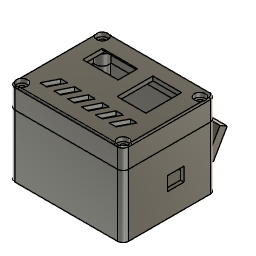
CaseCameraSlider (Autodesk Fusion 360 design; units mm, degrees)
Autodesk Fusion 360 part; units mm, degrees
note: some values were not read from the file. Set by a fixed rule: which face or edge a step refers to.
sketch "Schizzo3" plane through (0, 0, 0) normal (0, 0, 1) x (1, 0, 0)
  line L0 (0, 0) -> (80, 0)
  line L1 (80, 0) -> (80, -65)
  line L2 (80, -65) -> (0, -65)
  line L3 (0, -65) -> (0, 0)
  line L4 (81, -66) -> (-1, -66)
  line L5 (-1, -66) -> (-1, 1)
  line L6 (-1, 1) -> (81, 1)
  line L7 (81, 1) -> (81, -66)
  dimension "d8" = 80
  dimension "d9" = 65
  dimension "d10" = -1
  constraint horizontal L0
  constraint vertical L1
  constraint horizontal L2
  constraint vertical L3
  constraint coincident L0.start L3.end
  measures "d8" distance of L0.start L0.end
  measures "d9" distance of L0.start L2.end
extrude "Estrusione2" add sketch "Schizzo3" along normal blind 60 contours L0 L1 L2 L3 | L4 L5 L6 L7 makes body 1
sketch "Schizzo9" plane through (0, 0, 60) normal (0, 0, 1) x (-1, 0, 0)
  line L0 (-81, -1) -> (1, -1)
  line L1 (1, -1) -> (1, 66)
  line L2 (1, 66) -> (-81, 66)
  line L3 (-81, 66) -> (-81, -1)
  line L4 (1, -1) -> (-3.5, -1)
  line L5 (-3.5, -1) -> (-3.5, 3.5)
  line L6 (-3.5, 3.5) -> (1, 3.5)
  line L7 (1, 3.5) -> (1, -1)
  circle A0 centre (-3.5, 3.5) radius 4
  circle A1 centre (-3.5, 3.5) radius 2
  circle A2 centre (-76.5, 6.0015) radius 2
  circle A3 centre (-76.5, 6.0015) radius 4
  circle A4 centre (-3.5, 61.5) radius 2
  circle A5 centre (-3.5, 61.5) radius 4
  circle A6 centre (-76.5, 61.5) radius 2
  circle A7 centre (-76.5, 61.5) radius 4
  dimension "d70" = 4.5
  dimension "d71" = 4.5
  dimension "d72" = 8
  dimension "d73" = 4
  dimension "d81" = 8
  dimension "d82" = 4
  dimension "d86" = 8
  dimension "d87" = 4
  dimension "d88" = 8
  dimension "d89" = 4
  dimension "d90" = 4.5
  dimension "d91" = 4.5
  dimension "d92" = 4.5
  dimension "d93" = 4.5
  dimension "d94" = 4.5
  dimension "d95" = 4.5
  dimension "d96" = 4.5
  dimension "d97" = 4.5
  dimension "d98" = 4.5
  constraint horizontal L4
  constraint vertical L5
  constraint horizontal L6
  constraint vertical L7
  constraint coincident L0.end L1.start
  constraint coincident L5.end L6.start
  constraint concentric A0 A1
  constraint concentric A2 A3
  measures "d70" distance of L0.end L4.end
  measures "d71" distance of L0.end L6.end
  measures "d72" diameter of A0
  measures "d73" diameter of A1
  measures "d81" diameter of A3
  measures "d82" diameter of A2
  measures "d86" diameter of A5
  measures "d87" diameter of A4
  measures "d88" diameter of A7
  measures "d89" diameter of A6
  measures "d90" distance of L1 A4.centre
  measures "d91" distance of L1 A4.centre
  measures "d92" distance of L2 A4.centre
  measures "d93" distance of L2 A4.centre
  measures "d94" distance of L3 A2.centre
  measures "d95" distance of L3 A6.centre
  measures "d96" distance of L3 A6.centre
  measures "d97" distance of L2 A6.centre
  measures "d98" distance of L2 A6.centre
extrude "Estrusione9" cut sketch "Schizzo9" against normal blind 3 contours A3 bodies 1
extrude "Estrusione7" cut sketch "Schizzo9" against normal blind 3 contours L5 L6 A0 A1 | L5 L6 A0 A1 bodies 1
extrude "Estrusione8" cut 1 faces at (4.6392, -4.0006, 60) along direction (0, 0, -1) blind 20 on bodies 1 bodies 1
extrude "Estrusione10" cut sketch "Schizzo9" against normal blind 20 contours A2 bodies 1
extrude "Estrusione11" cut sketch "Schizzo9" against normal blind 3 contours A7 bodies 1
extrude "Estrusione12" cut sketch "Schizzo9" against normal blind 20 contours A6 bodies 1
extrude "Estrusione13" cut sketch "Schizzo9" against normal blind 3 contours A5 bodies 1
extrude "Estrusione14" cut sketch "Schizzo9" against normal blind 20 contours A4 bodies 1
fillet "Raccordo2" radius 4 4 edges at (-1, -66, 30) (81, -66, 30) (-1, 1, 30) (81, 1, 30) on bodies 1
ref_plane "Piano di lavoro2" through (40, -32.5, 45) normal (0, 0, 1) x (1, 0, 0)
split "Dividi2" by plane through (40, -32.5, 45) normal (0, 0, 1) bodies 1 makes body 2 at (28.6865, -24.4183, 60)
shell "Shell3" thickness 2.5 removed faces 1 at (28.2599, -24.0427, 45) on bodies 1
shell "Shell4" thickness 3 removed faces 1 at (28.2599, -24.0427, 45) on bodies 2
fillet "Raccordo3" radius 1 8 edges at (0.1716, -64.8284, 60) (-1, -32.5, 60) (0.1716, -0.1716, 60) (40, 1, 60) (79.8284, -0.1716, 60) (81, -32.5, 60) (79.8284, -64.8284, 60) (40, -66, 60) on bodies 2
sketch "Schizzo20" plane through (0, 1, 0) normal (0, 1, 0) x (-1, 0, 0)
  line L0 (-3, 45) -> (-77, 45)
  line L1 (-77, 45) -> (-77, 0)
  line L2 (-77, 0) -> (-3, 0)
  line L3 (-3, 0) -> (-3, 45)
  line L4 (-50, 22.0662) -> (-25, 22.0662)
  line L5 (-25, 22.0662) -> (-25, 12.0662)
  line L6 (-25, 12.0662) -> (-50, 12.0662)
  line L7 (-50, 12.0662) -> (-50, 22.0662)
  dimension "d178" = 10
  constraint horizontal L4
  constraint vertical L5
  constraint horizontal L6
  constraint vertical L7
  measures "d178" distance of L4.start L6.end
extrude "Estrusione28" add sketch "Schizzo20" along normal blind 15 contours L4 L5 L6 L7 bodies 1
sketch "Schizzo21" plane through (50, 0, 0) normal (1, 0, 0) x (0, 1, 0)
  line L0 (1, 22.0662) -> (1, 12.0662)
  line L1 (1, 12.0662) -> (16, 12.0662)
  line L2 (16, 12.0662) -> (16, 22.0662)
  line L3 (16, 22.0662) -> (1, 22.0662)
  line L4 (16, 22.0662) -> (10.2265, 12.0662)
  line L5 (16, 22.0662) -> (27.547, 22.0662) construction
  dimension "d325" = 120
  constraint horizontal L5
  constraint coincident L2.end L3.start
  constraint coincident L1 L4.end
  measures "d325" angle of L4 L5
extrude "Estrusione29" cut sketch "Schizzo21" against normal up to surface (25 mm away) contours L1 L2 L4 bodies 1
sketch "Schizzo28" plane through (0, 1, 0) normal (0, 1, 0) x (-1, 0, 0)
  line L0 (-70, 25) -> (-63, 25)
  line L1 (-63, 25) -> (-63, 15)
  line L2 (-63, 15) -> (-70, 15)
  line L3 (-70, 15) -> (-70, 25)
  dimension "d197" = 7
  dimension "d202" = 10
  constraint horizontal L0
  constraint vertical L1
  constraint horizontal L2
  constraint vertical L3
  measures "d197" distance of L0.start L0.end
  measures "d202" distance of L0.start L2.end
extrude "Estrusione35" cut sketch "Schizzo28" against normal up to surface (2.5 mm away) bodies 1
fillet "Raccordo11" radius 2 4 edges at (63, -0.25, 15) (70, -0.25, 15) (63, -0.25, 25) (70, -0.25, 25) on bodies 1
sketch "Schizzo34" plane through (0, 0, 2.5) normal (0, 0, 1) x (-1, 0, 0)
  arc A0 (-78.5, 3) -> (-77, 1.5) centre (-77, 3) ccw
  line L0 (-77, 1.5) -> (-3, 1.5)
  arc A1 (-3, 1.5) -> (-1.5, 3) centre (-3, 3) ccw
  line L1 (-1.5, 3) -> (-1.5, 62)
  arc A2 (-1.5, 62) -> (-3, 63.5) centre (-3, 62) ccw
  line L2 (-3, 63.5) -> (-77, 63.5)
  arc A3 (-77, 63.5) -> (-78.5, 62) centre (-77, 62) ccw
  line L3 (-78.5, 62) -> (-78.5, 3)
  line L4 (-75, 1.5) -> (-3, 1.5)
  line L5 (-76, 64) -> (-4, 64)
  circle A4 centre (-22.5, 6) radius 1.5
  circle A5 centre (-72, 6) radius 1.5
  circle A6 centre (-72, 58.5) radius 1.5
  circle A7 centre (-72, 36.5) radius 1.5
  circle A8 centre (-6, 58.5) radius 1.5
  circle A9 centre (-6, 58.5) radius 3
  circle A10 centre (-72, 58.5) radius 3
  circle A11 centre (-72, 36.5) radius 3
  circle A12 centre (-72, 6) radius 3
  circle A13 centre (-22.5, 6) radius 3
  point P0 (-40, 34.5)
  dimension "d274" = 72
  dimension "d279" = 3
  dimension "d280" = 3
  dimension "d281" = 3
  dimension "d282" = 3
  dimension "d283" = 3
  dimension "d294" = 6
  dimension "d295" = 6
  dimension "d296" = 6
  dimension "d297" = 6
  dimension "d298" = 6
  constraint horizontal L5
  constraint concentric A8 A9
  constraint concentric A6 A10
  constraint concentric A7 A11
  constraint concentric A5 A12
  constraint concentric A4 A13
  measures "d274" distance of L4.start L0.end
  measures "d279" diameter of A4
  measures "d280" diameter of A5
  measures "d281" diameter of A6
  measures "d282" diameter of A7
  measures "d283" diameter of A8
  measures "d294" diameter of A9
  measures "d295" diameter of A10
  measures "d296" diameter of A11
  measures "d297" diameter of A12
  measures "d298" diameter of A13
extrude "Estrusione48" add sketch "Schizzo34" along normal blind 4 contours A9 | A10 | A11 | A12 | A13 bodies 1
sketch "Schizzo35" plane through (1.5, 0, 0) normal (1, 0, 0) x (0, 1, 0)
  line L0 (-57.4689, 45) -> (-57.4689, 37.5)
  line L1 (-57.4689, 37.5) -> (-62, 37.5)
  line L2 (-62, 37.5) -> (-62, 2.5)
  line L3 (-62, 2.5) -> (-3, 2.5)
  line L4 (-3, 2.5) -> (-3, 37.5)
  line L5 (-3, 37.5) -> (-7.5311, 37.5)
  line L6 (-7.5311, 37.5) -> (-7.5311, 45)
  line L7 (-7.5311, 45) -> (-57.4689, 45)
sketch "Schizzo36" plane through (-1, 0, 0) normal (-1, 0, 0) x (0, -1, 0)
  line L0 (62, 45) -> (3, 45)
  line L1 (3, 45) -> (3, 0)
  line L2 (3, 0) -> (62, 0)
  line L3 (62, 0) -> (62, 45)
  line L4 (5, 16.5) -> (15, 16.5)
  line L5 (15, 16.5) -> (15, 6.5)
  line L6 (15, 6.5) -> (5, 6.5)
  line L7 (5, 6.5) -> (5, 16.5)
  point P0 (32.5, 23.8824)
  dimension "d305" = 10
  dimension "d306" = 10
  dimension "d324" = 2
  constraint horizontal L4
  constraint vertical L5
  constraint horizontal L6
  constraint vertical L7
  measures "d305" distance of L4.start L4.end
  measures "d306" distance of L4.start L6.end
  measures "d324" distance of L1 L7
extrude "Estrusione49" cut sketch "Schizzo36" against normal blind 2.5 contours L4 L5 L6 L7 bodies 1
sketch "Schizzo41" plane through (81, 0, 0) normal (1, 0, 0) x (0, 1, 0)
  line L0 (-3, 45) -> (-62, 45)
  line L1 (-62, 45) -> (-62, 0)
  line L2 (-62, 0) -> (-3, 0)
  line L3 (-3, 0) -> (-3, 45)
  line L4 (-22, 17) -> (-34, 17)
  line L5 (-34, 17) -> (-34, 27)
  line L6 (-34, 27) -> (-22, 27)
  line L7 (-22, 27) -> (-22, 17)
  point P0 (-28, 22)
  dimension "d312" = 12
  dimension "d313" = 10
  dimension "d315" = 18
  dimension "d316" = 25
  constraint horizontal L4
  constraint vertical L5
  constraint horizontal L6
  constraint vertical L7
  measures "d312" distance of L4.start L4.end
  measures "d313" distance of L4.start L6.end
  measures "d315" distance of L0 L6
  measures "d316" distance of L3 P0
extrude "Estrusione50" cut sketch "Schizzo41" against normal up to surface (2.5 mm away) contours L4 L5 L6 L7 bodies 1
sketch "Schizzo43" plane through (0, 2.445, -1.4116) normal (0, 0.866025, -0.5) x (-1, 0, 0)
  line L0 (-25, 15.5629) -> (-25, 27.1099)
  line L1 (-25, 27.1099) -> (-50, 27.1099)
  line L2 (-50, 27.1099) -> (-50, 15.5629)
  line L3 (-50, 15.5629) -> (-25, 15.5629)
  line L4 (-7, 11) -> (-67, 11)
  line L5 (-67, 11) -> (-67, 31)
  line L6 (-67, 31) -> (-7, 31)
  line L7 (-7, 31) -> (-7, 11)
  line L8 (-7, 11) -> (-67, 31) construction
  line L9 (-67, 11) -> (-7, 31) construction
  point P0 (-37, 21)
  dimension "d326" = 60
  dimension "d327" = 20
  constraint horizontal L4
  constraint perpendicular L4 L5
  constraint parallel L4 L6
  constraint parallel L5 L7
  constraint coincident L8 P0
  constraint coincident L9 P0
  measures "d326" distance of L5.end L6.end
  measures "d327" distance of L4.end L5.end
extrude "Estrusione51" add sketch "Schizzo43" along normal blind 6 contours L0 L1 L2 L3 | L4 L5 L6 L7 bodies 1
sketch "Schizzo44" plane through (0, 2.445, -1.4116) normal (0, -0.866025, 0.5) x (1, 0, 0)
  line L0 (67, 31) -> (7, 31)
  line L1 (7, 31) -> (7, 11)
  line L2 (7, 11) -> (67, 11)
  line L3 (67, 11) -> (67, 31)
  line L4 (25, 15.5629) -> (25, 27.1099)
  line L5 (25, 27.1099) -> (50, 27.1099)
  line L6 (50, 27.1099) -> (50, 15.5629)
  circle A0 centre (15, 21) radius 2.5
  circle A1 centre (15, 21) radius 5
  circle A2 centre (59, 20.998) radius 2.5
  circle A3 centre (59, 20.998) radius 5
  line L7 (50, 15.5629) -> (25, 15.5629)
  line L8 (67, 21) -> (7, 21)
  dimension "d330" = 5
  dimension "d331" = 10
  dimension "d332" = 8
  dimension "d333" = 5
  dimension "d334" = 10
  dimension "d335" = 8
  dimension "d340" = 60
  constraint concentric A0 A1
  constraint concentric A2 A3
  constraint midpoint L3 L8.start
  constraint midpoint L1 L8.end
  measures "d330" diameter of A0
  measures "d331" diameter of A1
  measures "d332" distance of L1 A0.centre
  measures "d333" diameter of A2
  measures "d334" diameter of A3
  measures "d335" distance of L3 A2.centre
  measures "d340" distance of L8.start L8.end
extrude "Estrusione52" cut sketch "Schizzo44" against normal up to surface (6 mm away) contours A2 L8 | A2 L8 | A0 L8 | A0 L8 bodies 1
sketch "Schizzo45" plane through (0, 0, 2.5) normal (0, 0, 1) x (-1, 0, 0)
  circle A0 centre (-22.5, 6) radius 3
  circle A1 centre (-72, 6) radius 3
  arc A2 (-78.5, 3) -> (-77, 1.5) centre (-77, 3) ccw
  line L0 (-77, 1.5) -> (-3, 1.5)
  arc A3 (-3, 1.5) -> (-1.5, 3) centre (-3, 3) ccw
  line L1 (-1.5, 3) -> (-1.5, 62)
  arc A4 (-1.5, 62) -> (-3, 63.5) centre (-3, 62) ccw
  line L2 (-3, 63.5) -> (-77, 63.5)
  arc A5 (-77, 63.5) -> (-78.5, 62) centre (-77, 62) ccw
  line L3 (-78.5, 62) -> (-78.5, 3)
  circle A6 centre (-72, 36.5) radius 3
  circle A7 centre (-72, 58.5) radius 3
  circle A8 centre (-6, 58.5) radius 3
  line L4 (-20, 20) -> (-30, 20)
  line L5 (-30, 20) -> (-30, 50)
  line L6 (-30, 50) -> (-20, 50)
  line L7 (-20, 50) -> (-20, 20)
  line L8 (-50, 20) -> (-60, 20)
  line L9 (-60, 20) -> (-60, 50)
  line L10 (-60, 50) -> (-50, 50)
  line L11 (-50, 50) -> (-50, 20)
  constraint horizontal L4
  constraint vertical L5
  constraint horizontal L6
  constraint vertical L7
  constraint horizontal L8
  constraint vertical L9
  constraint horizontal L10
  constraint vertical L11
extrude "Estrusione54" cut sketch "Schizzo45" against normal up to surface (2.5 mm away) contours L4 L5 L6 L7 | L8 L9 L10 L11 bodies 1
sketch "Schizzo29" plane through (0, 0, 60) normal (0, 0, 1) x (-1, 0, 0)
  line L0 (0, 5.4365) -> (0, 59.5635)
  arc A0 (-5.4365, 65) -> (0, 59.5635) centre (-3.5, 61.5) ccw
  line L1 (-5.4365, 65) -> (-74.5635, 65)
  arc A1 (-80, 59.5635) -> (-74.5635, 65) centre (-76.5, 61.5) ccw
  line L2 (-80, 59.5635) -> (-80, 7.938)
  arc A2 (-80, 4.065) -> (-80, 7.938) centre (-76.5, 6.0015) ccw
  arc A3 (-80, 3) -> (-77, 0) centre (-77, 3) ccw
  line L3 (-77, 0) -> (-5.4365, 0)
  arc A4 (0, 5.4365) -> (-5.4365, 0) centre (-3.5, 3.5) ccw
  line L4 (-10, 45) -> (-70, 45)
  line L5 (-70, 45) -> (-70, 55)
  line L6 (-70, 55) -> (-10, 55)
  line L7 (-10, 55) -> (-10, 45)
  line L8 (-10, 55) -> (-15, 45)
  line L9 (-20, 45) -> (-15, 55)
  line L10 (-25, 45) -> (-20, 55)
  line L11 (-30, 45) -> (-25, 55)
  line L12 (-35, 45) -> (-30, 55)
  line L13 (-70, 45) -> (-65.0034, 55)
  line L14 (-40, 45) -> (-35, 55)
  line L15 (-44.9844, 45) -> (-40, 55)
  line L16 (-50.0578, 45) -> (-45.1322, 55)
  line L17 (-54.9341, 45) -> (-50.0085, 55)
  line L18 (-60.2537, 45) -> (-55, 55)
  line L19 (-65.1793, 45) -> (-59.9256, 55)
  line L20 (-80, 4.065) -> (-80, 3)
  constraint horizontal L4
  constraint vertical L5
  constraint horizontal L6
  constraint vertical L7
  constraint coincident L4 L8.end
  constraint coincident L4 L9.start
  constraint parallel L8 L9
  constraint coincident L4 L10.start
  constraint coincident L6 L10.end
  constraint parallel L9 L10
  constraint coincident L4 L11.start
  constraint coincident L6 L11.end
  constraint parallel L10 L11
  constraint coincident L4 L12.start
  constraint coincident L6 L12.end
  constraint parallel L11 L12
  constraint coincident L6 L13.end
  constraint midpoint L4 L14.start
  constraint coincident L6 L14.end
  constraint parallel L12 L14
  constraint coincident L4 L15.start
  constraint midpoint L6 L15.end
  constraint coincident L4 L16.start
  constraint coincident L6 L16.end
  constraint coincident L4 L17.start
  constraint coincident L6 L17.end
  constraint parallel L16 L17
  constraint coincident L4 L18.start
  constraint coincident L6 L18.end
  constraint coincident L4 L19.start
  constraint coincident L6 L19.end
  constraint parallel L18 L19
extrude "Estrusione36" cut sketch "Schizzo29" against normal up to surface (3 mm away) contours L4 L6 L8 L9 | L4 L6 L10 L11 | L4 L6 L12 L14 | L4 L6 L15 L16 | L4 L6 L17 L18 | L4 L6 L13 L19 bodies 2
sketch "Schizzo30" plane through (0, 0, 60) normal (0, 0, 1) x (-1, 0, 0)
  line L0 (-44.9844, 45) -> (-50.0578, 45)
  line L1 (-50.0578, 45) -> (-45.1322, 55)
  line L2 (-45.1322, 55) -> (-40, 55)
  line L3 (-40, 55) -> (-44.9844, 45)
  line L4 (-20, 45) -> (-15, 55)
  line L5 (-15, 55) -> (-10, 55)
  line L6 (-10, 55) -> (-15, 45)
  line L7 (-15, 45) -> (-20, 45)
  line L8 (-54.9341, 45) -> (-60.2537, 45)
  line L9 (-60.2537, 45) -> (-55, 55)
  line L10 (-55, 55) -> (-50.0085, 55)
  line L11 (-50.0085, 55) -> (-54.9341, 45)
  line L12 (-35, 45) -> (-40, 45)
  line L13 (-40, 45) -> (-35, 55)
  line L14 (-35, 55) -> (-30, 55)
  line L15 (-30, 55) -> (-35, 45)
  line L16 (-25, 45) -> (-30, 45)
  line L17 (-30, 45) -> (-25, 55)
  line L18 (-25, 55) -> (-20, 55)
  line L19 (-20, 55) -> (-25, 45)
  line L20 (-70, 45) -> (-65.0034, 55)
  line L21 (-65.0034, 55) -> (-59.9256, 55)
  line L22 (-59.9256, 55) -> (-65.1793, 45)
  line L23 (-65.1793, 45) -> (-70, 45)
  line L24 (0, 5.4365) -> (0, 59.5635)
  arc A0 (-5.4365, 65) -> (0, 59.5635) centre (-3.5, 61.5) ccw
  line L25 (-5.4365, 65) -> (-74.5635, 65)
  arc A1 (-80, 59.5635) -> (-74.5635, 65) centre (-76.5, 61.5) ccw
  line L26 (-80, 59.5635) -> (-80, 7.938)
  arc A2 (-80, 4.065) -> (-80, 7.938) centre (-76.5, 6.0015) ccw
  arc A3 (-80, 3) -> (-77, 0) centre (-77, 3) ccw
  line L27 (-77, 0) -> (-5.4365, 0)
  arc A4 (0, 5.4365) -> (-5.4365, 0) centre (-3.5, 3.5) ccw
  line L28 (-80, 4.065) -> (-80, 3)
  line L29 (-11, 11) -> (-36.4, 11)
  line L30 (-36.4, 11) -> (-36.4, 25)
  line L31 (-36.4, 25) -> (-11, 25)
  line L32 (-11, 25) -> (-11, 11)
  dimension "d344" = 25.4
  dimension "d345" = 14
  constraint horizontal L29
  constraint vertical L30
  constraint horizontal L31
  constraint vertical L32
  measures "d344" distance of L29.start L29.end
  measures "d345" distance of L29.start L31.end
extrude "Estrusione55" cut sketch "Schizzo30" against normal up to surface (3 mm away) contours L29 L30 L31 L32 bodies 2
sketch "Schizzo46" plane through (0, 0, 57) normal (0, 0, -1) x (1, 0, 0)
  line L0 (11, 11) -> (11, 25)
  line L1 (11, 25) -> (36.4, 25)
  line L2 (36.4, 25) -> (36.4, 11)
  line L3 (36.4, 11) -> (11, 11)
  line L4 (50.0578, 45) -> (44.9844, 45)
  line L5 (44.9844, 45) -> (40, 55)
  line L6 (40, 55) -> (45.1322, 55)
  line L7 (45.1322, 55) -> (50.0578, 45)
  line L8 (15, 55) -> (20, 45)
  line L9 (20, 45) -> (15, 45)
  line L10 (15, 45) -> (10, 55)
  line L11 (10, 55) -> (15, 55)
  line L12 (60.2537, 45) -> (54.9341, 45)
  line L13 (54.9341, 45) -> (50.0085, 55)
  line L14 (50.0085, 55) -> (55, 55)
  line L15 (55, 55) -> (60.2537, 45)
  line L16 (40, 45) -> (35, 45)
  line L17 (35, 45) -> (30, 55)
  line L18 (30, 55) -> (35, 55)
  line L19 (35, 55) -> (40, 45)
  line L20 (30, 45) -> (25, 45)
  line L21 (25, 45) -> (20, 55)
  line L22 (20, 55) -> (25, 55)
  line L23 (25, 55) -> (30, 45)
  line L24 (65.0034, 55) -> (70, 45)
  line L25 (70, 45) -> (65.1793, 45)
  line L26 (65.1793, 45) -> (59.9256, 55)
  line L27 (59.9256, 55) -> (65.0034, 55)
  arc A0 (2, 54.6626) -> (10.3374, 63) centre (3.5, 61.5) ccw
  line L28 (2, 54.6626) -> (2, 10.3374)
  arc A1 (10.3374, 2) -> (2, 10.3374) centre (3.5, 3.5) ccw
  line L29 (10.3374, 2) -> (70.7565, 2)
  arc A2 (78, 12.8389) -> (70.7565, 2) centre (76.5, 6.0015) ccw
  line L30 (78, 12.8389) -> (78, 54.6626)
  arc A3 (69.6626, 63) -> (78, 54.6626) centre (76.5, 61.5) ccw
  line L31 (69.6626, 63) -> (10.3374, 63)
  line L32 (36.4, 31.05) -> (11, 31.05)
  line L33 (11, 31.05) -> (11, 4.95)
  line L34 (11, 4.95) -> (36.4, 4.95)
  line L35 (36.4, 4.95) -> (36.4, 31.05)
  line L36 (36.4, 31.05) -> (11, 4.95) construction
  line L37 (11, 31.05) -> (36.4, 4.95) construction
  point P0 (23.7, 18)
  dimension "d348" = 25.4
  dimension "d349" = 26.1
  constraint horizontal L32
  constraint perpendicular L32 L33
  constraint parallel L32 L34
  constraint parallel L33 L35
  constraint coincident L36 P0
  constraint coincident L37 P0
  measures "d348" distance of L33.end L34.end
  measures "d349" distance of L32.end L33.end
extrude "Estrusione56" cut sketch "Schizzo46" against normal blind 2 contours L3 L33 L34 L35 | L1 L32 L33 L35 bodies 2
sketch "Schizzo47" plane through (0, 0, 59) normal (0, 0, -1) x (1, 0, 0)
  line L0 (36.4, 4.95) -> (36.4, 11)
  line L1 (36.4, 11) -> (11, 11)
  line L2 (11, 11) -> (11, 4.95)
  line L3 (11, 4.95) -> (36.4, 4.95)
  circle A0 centre (12.7, 7.25) radius 1
  circle A1 centre (34.7, 7.25) radius 1
  circle A2 centre (34.7, 28.75) radius 1
  circle A3 centre (12.7, 28.75) radius 1
  line L4 (11, 4.95) -> (11, 31.05)
  line L5 (36.4, 31.05) -> (36.4, 4.95)
  line L6 (11, 31.05) -> (36.4, 31.05)
  circle A4 centre (12.7, 28.75) radius 2
  circle A5 centre (34.7, 28.75) radius 2
  circle A6 centre (34.7, 7.25) radius 2
  circle A7 centre (12.7, 7.25) radius 2
  dimension "d352" = 2
  dimension "d353" = 2
  dimension "d355" = 1.7
  dimension "d356" = 1.7
  dimension "d357" = 2.3
  dimension "d358" = 2.3
  dimension "d359" = 2
  dimension "d360" = 2
  dimension "d361" = 1.7
  dimension "d362" = 1.7
  dimension "d363" = 2.3
  dimension "d364" = 2.3
  dimension "d365" = 4
  dimension "d366" = 4
  dimension "d367" = 4
  dimension "d368" = 4
  constraint concentric A3 A4
  constraint concentric A2 A5
  constraint concentric A1 A6
  constraint concentric A0 A7
  measures "d352" diameter of A0
  measures "d353" diameter of A1
  measures "d355" distance of L0 A1.centre
  measures "d356" distance of L2 A0.centre
  measures "d357" distance of L3 A1.centre
  measures "d358" distance of L3 A0.centre
  measures "d359" diameter of A2
  measures "d360" diameter of A3
  measures "d361" distance of A3.centre L4
  measures "d362" distance of A2.centre L5
  measures "d363" distance of A2.centre L6
  measures "d364" distance of A3.centre L6
  measures "d365" diameter of A4
  measures "d366" diameter of A5
  measures "d367" diameter of A6
  measures "d368" diameter of A7
extrude "Estrusione57" add sketch "Schizzo47" along normal blind 2 contours L0 L5 A6 | L0 L5 A6 | L2 L4 A7 | L2 L4 A7 | L5 A5 | L5 A5 | L4 A4 | L4 A4 bodies 2
sketch "Schizzo48" plane through (0, 0, 60) normal (0, 0, 1) x (-1, 0, 0)
  line L0 (-11, 25) -> (-11, 11)
  line L1 (-11, 11) -> (-36.4, 11)
  line L2 (-36.4, 11) -> (-36.4, 25)
  line L3 (-36.4, 25) -> (-11, 25)
  line L4 (-44.9844, 45) -> (-50.0578, 45)
  line L5 (-50.0578, 45) -> (-45.1322, 55)
  line L6 (-45.1322, 55) -> (-40, 55)
  line L7 (-40, 55) -> (-44.9844, 45)
  line L8 (-20, 45) -> (-15, 55)
  line L9 (-15, 55) -> (-10, 55)
  line L10 (-10, 55) -> (-15, 45)
  line L11 (-15, 45) -> (-20, 45)
  line L12 (-54.9341, 45) -> (-60.2537, 45)
  line L13 (-60.2537, 45) -> (-55, 55)
  line L14 (-55, 55) -> (-50.0085, 55)
  line L15 (-50.0085, 55) -> (-54.9341, 45)
  line L16 (-35, 45) -> (-40, 45)
  line L17 (-40, 45) -> (-35, 55)
  line L18 (-35, 55) -> (-30, 55)
  line L19 (-30, 55) -> (-35, 45)
  line L20 (-25, 45) -> (-30, 45)
  line L21 (-30, 45) -> (-25, 55)
  line L22 (-25, 55) -> (-20, 55)
  line L23 (-20, 55) -> (-25, 45)
  line L24 (-70, 45) -> (-65.0034, 55)
  line L25 (-65.0034, 55) -> (-59.9256, 55)
  line L26 (-59.9256, 55) -> (-65.1793, 45)
  line L27 (-65.1793, 45) -> (-70, 45)
  line L28 (0, 5.4365) -> (0, 59.5635)
  arc A0 (-5.4365, 65) -> (0, 59.5635) centre (-3.5, 61.5) ccw
  line L29 (-5.4365, 65) -> (-74.5635, 65)
  arc A1 (-80, 59.5635) -> (-74.5635, 65) centre (-76.5, 61.5) ccw
  line L30 (-80, 59.5635) -> (-80, 7.938)
  arc A2 (-80, 4.065) -> (-80, 7.938) centre (-76.5, 6.0015) ccw
  line L31 (-80, 4.065) -> (-80, 3)
  arc A3 (-80, 3) -> (-77, 0) centre (-77, 3) ccw
  line L32 (-77, 0) -> (-5.4365, 0)
  arc A4 (0, 5.4365) -> (-5.4365, 0) centre (-3.5, 3.5) ccw
  line L33 (-45, 10) -> (-65.7, 10)
  line L34 (-65.7, 10) -> (-65.7, 35.7)
  line L35 (-65.7, 35.7) -> (-45, 35.7)
  line L36 (-45, 35.7) -> (-45, 10)
  dimension "d371" = 20.7
  dimension "d372" = 25.7
  constraint horizontal L33
  constraint vertical L34
  constraint horizontal L35
  constraint vertical L36
  measures "d371" distance of L33.start L33.end
  measures "d372" distance of L33.start L35.end
extrude "Estrusione58" cut sketch "Schizzo48" against normal up to surface (3 mm away) contours L33 L34 L35 L36 bodies 2
sketch "Schizzo49" plane through (0, 0, 57) normal (0, 0, -1) x (1, 0, 0)
  line L0 (45, 10) -> (45, 35.7)
  line L1 (45, 35.7) -> (65.7, 35.7)
  line L2 (65.7, 35.7) -> (65.7, 10)
  line L3 (65.7, 10) -> (45, 10)
  line L4 (36.4, 31.05) -> (36.4, 29.8036)
  line L5 (36.4, 4.95) -> (11, 4.95)
  line L6 (11, 8.3036) -> (11, 27.6964)
  line L7 (11, 31.05) -> (36.4, 31.05)
  line L8 (50.0578, 45) -> (44.9844, 45)
  line L9 (44.9844, 45) -> (40, 55)
  line L10 (40, 55) -> (45.1322, 55)
  line L11 (45.1322, 55) -> (50.0578, 45)
  line L12 (15, 55) -> (20, 45)
  line L13 (20, 45) -> (15, 45)
  line L14 (15, 45) -> (10, 55)
  line L15 (10, 55) -> (15, 55)
  line L16 (60.2537, 45) -> (54.9341, 45)
  line L17 (54.9341, 45) -> (50.0085, 55)
  line L18 (50.0085, 55) -> (55, 55)
  line L19 (55, 55) -> (60.2537, 45)
  line L20 (40, 45) -> (35, 45)
  line L21 (35, 45) -> (30, 55)
  line L22 (30, 55) -> (35, 55)
  line L23 (35, 55) -> (40, 45)
  line L24 (30, 45) -> (25, 45)
  line L25 (25, 45) -> (20, 55)
  line L26 (20, 55) -> (25, 55)
  line L27 (25, 55) -> (30, 45)
  line L28 (65.0034, 55) -> (70, 45)
  line L29 (70, 45) -> (65.1793, 45)
  line L30 (65.1793, 45) -> (59.9256, 55)
  line L31 (59.9256, 55) -> (65.0034, 55)
  arc A0 (2, 54.6626) -> (10.3374, 63) centre (3.5, 61.5) ccw
  line L32 (2, 54.6626) -> (2, 10.3374)
  arc A1 (10.3374, 2) -> (2, 10.3374) centre (3.5, 3.5) ccw
  line L33 (10.3374, 2) -> (70.7565, 2)
  arc A2 (78, 12.8389) -> (70.7565, 2) centre (76.5, 6.0015) ccw
  line L34 (78, 12.8389) -> (78, 54.6626)
  arc A3 (69.6626, 63) -> (78, 54.6626) centre (76.5, 61.5) ccw
  line L35 (69.6626, 63) -> (10.3374, 63)
  circle A4 centre (69.85, 12.15) radius 1.5
  circle A5 centre (43.35, 12.45) radius 1.5
  circle A6 centre (43.35, 33.25) radius 1.5
  circle A7 centre (69.85, 33.55) radius 1.5
  line L36 (38.35, 36.05) -> (72.35, 36.05)
  line L37 (72.35, 36.05) -> (72.35, 9.65)
  line L38 (72.35, 9.65) -> (38.35, 9.65)
  line L39 (38.35, 9.65) -> (38.35, 36.05)
  line L40 (38.35, 36.05) -> (72.35, 9.65) construction
  line L41 (72.35, 36.05) -> (38.35, 9.65) construction
  circle A8 centre (12.7, 7.25) radius 1
  circle A9 centre (34.7, 7.25) radius 1
  arc A10 (11, 27.6964) -> (11, 29.8036) centre (12.7, 28.75) ccw
  line L42 (11, 29.8036) -> (11, 31.05)
  arc A11 (36.4, 29.8036) -> (36.4, 27.6964) centre (34.7, 28.75) ccw
  line L43 (36.4, 27.6964) -> (36.4, 8.3036)
  arc A12 (36.4, 8.3036) -> (36.4, 6.1964) centre (34.7, 7.25) ccw
  line L44 (36.4, 6.1964) -> (36.4, 4.95)
  line L45 (11, 4.95) -> (11, 6.1964)
  arc A13 (11, 6.1964) -> (11, 8.3036) centre (12.7, 7.25) ccw
  circle A14 centre (34.7, 28.75) radius 1
  circle A15 centre (12.7, 28.75) radius 1
  point P0 (55.35, 22.85)
  point P1 (55.35, 22.85)
  dimension "d379" = 3
  dimension "d380" = 3
  dimension "d382" = 3
  dimension "d383" = 3
  dimension "d385" = 34
  dimension "d386" = 26.4
  dimension "d387" = 2.5
  dimension "d388" = 2.5
  dimension "d389" = 2.5
  dimension "d390" = 2.5
  dimension "d391" = 2.8
  dimension "d392" = 5
  dimension "d393" = 5
  dimension "d394" = 2.8
  constraint horizontal L36
  constraint perpendicular L36 L37
  constraint parallel L36 L38
  constraint parallel L37 L39
  constraint coincident L40 P1
  constraint coincident L41 P1
  constraint coincident P1 P0
  measures "d379" diameter of A4
  measures "d380" diameter of A5
  measures "d382" diameter of A6
  measures "d383" diameter of A7
  measures "d385" distance of L37.end L38.end
  measures "d386" distance of L36.end L37.end
  measures "d387" distance of A4.centre L37
  measures "d388" distance of A4.centre L38
  measures "d389" distance of A7.centre L37
  measures "d390" distance of A7.centre L36
  measures "d391" distance of A6.centre L36
  measures "d392" distance of A6.centre L39
  measures "d393" distance of A5.centre L39
  measures "d394" distance of A5.centre L38
extrude "Estrusione60" cut sketch "Schizzo49" against normal blind 2 contours A4 | A5 | A6 | A7 bodies 2
extrude "Estrusione61" add 1 faces at (45, -27.1333, 59) along direction (1, 0, 0) blind 1.5 on bodies 2 bodies 2
extrude "Estrusione62" cut 1 faces at (65.7, -18.5667, 59) along direction (1, 0, 0) blind 1.5 on bodies 2 bodies 2
